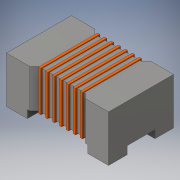
# Autodesk Inventor part: DLW21H_CM_Choke
Saved by Autodesk Inventor 2016 (Build 200138000, 138)
## iProperties
Created: 2017-03-04
Part Number: DLW21H_CM_Choke
Material: Generic
Document SubType Name: Modeling
Designer: jfixelle
Density: 1 g/cm^3
Appearance: Smooth - Medium Gray
Author: jfixelle
Autodesk Inventor part; units mm, degrees
ref_plane "YZ Plane" through (0, 0, 0) normal (1, 0, 0) x (0, 1, 0)
ref_plane "XZ Plane" through (0, 0, 0) normal (0, 1, 0) x (-1, 0, 0)
ref_plane "XY Plane" through (0, 0, 0) normal (0, 0, 1) x (1, 0, 0)
sketch "Sketch1" plane through (0, 0, 0) normal (0, 1, 0) x (-1, 0, 0)
  line L0 (1.1, 0.7) -> (-1.1, 0.7)
  line L1 (-1.1, 0.7) -> (-1.1, -0.7)
  line L2 (-1.1, -0.7) -> (1.1, -0.7)
  line L3 (1.1, -0.7) -> (1.1, 0.7)
  line L4 (-0.6, 0.7) -> (-0.6, -0.7)
  line L5 (0.6, 0.7) -> (0.6, -0.7)
  line L6 (0.6, 0.6) -> (-0.6, 0.6)
  line L7 (0.6, -0.6) -> (-0.6, -0.6)
  line L8 (-0.6, 0.7) -> (-0.5, 0.6)
  line L9 (0.6, 0.7) -> (0.5, 0.6)
  line L10 (0.6, -0.7) -> (0.5, -0.6)
  line L11 (-0.6, -0.7) -> (-0.5, -0.6)
  point P0 (0, 0)
  dimension "d0" = 1.4
  dimension "d1" = 0.7
  dimension "d2" = 2.2
  dimension "d3" = 1.1
  dimension "d4" = 0.5
  dimension "d5" = 0.5
  dimension "d6" = 0.6
  dimension "d7" = 0.6
  dimension "d8" = 45
  dimension "d9" = 45
  dimension "d10" = 45
  constraints: 24 end point, 12 point on line, 5 perpendicular, 3 parallel, 1 horizontal
  measures "d0" distance of L2.end L0.start
  measures "d1" distance from line of point (0, 0) L2
  measures "d2" distance of L1.end L2.end
  measures "d3" distance from line of point (0, 0) L3
  measures "d4" distance between parallel lines of L5 L3
  measures "d5" distance between parallel lines of L1 L4
  measures "d6" distance from line of L7 point (0, 0)
  measures "d7" distance from line of point (0, 0) L6
  measures "d8" angle of L6 L9
  measures "d9" angle of L7 L10
  measures "d10" angle of L7 L11
extrude "Extrusion1" add sketch "Sketch1" along normal blind 0.83 contours L3 L2 L5 L0 | L5 L6 L9 | L4 L2 L1 L0 | L8 L6 L4 | L5 L7 L4 L6 | L10 L7 L5 | L4 L7 L11
sketch "Sketch2" plane through (0, 0, 0) normal (0, -1, 0) x (1, 0, 0)
  line L0 (1.1, -0.7) -> (0.6, -0.7) projected
  line L1 (1.1, -0.7) -> (0.65, -0.7)
  line L2 (0.65, -0.7) -> (0.65, -0.3)
  line L3 (0.65, -0.3) -> (1.1, -0.3)
  line L4 (1.1, -0.3) -> (1.1, -0.7)
  point P0 (0, 0)
  dimension "d13" = 0.4
  dimension "d14" = 0.45
  constraints: 8 end point, 2 parallel, 1 horizontal, 1 perpendicular
  measures "d13" distance of L1.end L2.end
  measures "d14" distance of L2.end L3.end
extrude "Extrusion2" add sketch "Sketch2" along normal blind 0.17
mirror "Mirror1" about plane through (0, 0, 0) normal (1, 0, 0) of "Extrusion2"
mirror "Mirror2" about plane through (0, 0, 0) normal (0, 0, 1) of "Extrusion2", "Mirror1"
sketch "Sketch3" plane through (0, 0, 0) normal (1, 0, 0) x (0, 1, 0)
  line L0 (-0.0201, -0.6354) -> (0.8484, -0.6354)
  line L1 (0.8484, -0.6354) -> (0.8484, 0)
  line L2 (0.8484, 0) -> (-0.0201, 0)
  line L3 (-0.0201, 0) -> (-0.0201, -0.6354)
  line L4 (-0.0201, 0.6354) -> (0.8484, 0.6354)
  line L5 (0.8484, 0.6354) -> (0.8484, 0)
  line L6 (-0.0201, 0) -> (-0.0201, 0.6354)
  point P0 (0, 0)
  constraints: 14 end point, 2 parallel, 2 symmetric about line, 1 horizontal, 1 perpendicular
extrude "Extrusion3" add sketch "Sketch3" along normal mid plane 0.05
pattern_linear "Rectangular Pattern1" count 7 spacing 0.15 along (1, 0, 0) of "Extrusion3" first direction both ways yes
body "Solid1"
